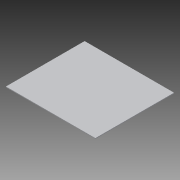
# Autodesk Inventor part: Cuarto
Saved by Autodesk Inventor 2013 (Build 170138000, 138)
## iProperties
Created: 2015-11-12
Part Number: Cuarto
Material: Generic
Document SubType Name: Modeling
Designer: serge
Density: 1 g/cm^3
Author: serge
Autodesk Inventor part; units mm, degrees
ref_plane "YZ Plane" through (0, 0, 0) normal (1, 0, 0) x (0, 1, 0)
ref_plane "XZ Plane" through (0, 0, 0) normal (0, 1, 0) x (-1, 0, 0)
ref_plane "XY Plane" through (0, 0, 0) normal (0, 0, 1) x (1, 0, 0)
sketch "Sketch1" plane through (0, 0, 0) normal (0, 0, 1) x (1, 0, 0)
  line L0 (-28.239, -20.7889) -> (2407.6723, -20.7889)
  line L1 (2407.6723, -20.7889) -> (2407.6723, 2122.0559)
  line L2 (2407.6723, 2122.0559) -> (-28.239, 2122.0559)
  line L3 (-28.239, 2122.0559) -> (-28.239, -20.7889)
  point P0 (0, 0)
  constraints: 8 end point, 2 parallel, 1 horizontal, 1 perpendicular
extrude "Extrusion1" add sketch "Sketch1" along normal blind 20
body "Solid1"
